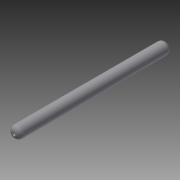
# Autodesk Inventor part: Pool Noodle Part2 (26x28 robot)
Saved by Autodesk Inventor 2014 SP1 (Build 180222100, 222)
## iProperties
Created: 2013-01-06
Part Number: Pool Noodle Part2 (26x28 robot)
Material: Generic
Document SubType Name: Modeling
Designer: Moses
Density: 0.0258246 g/cm^3
Mass: 45.1324 g
Surface Area: 1630.33 cm^2
Volume: 1747.66 cm^3
Appearance: Default
Author: Moses
Autodesk Inventor part; units mm, degrees
ref_plane "YZ Plane" through (0, 0, 0) normal (1, 0, 0) x (0, 1, 0)
ref_plane "XZ Plane" through (0, 0, 0) normal (0, 1, 0) x (-1, 0, 0)
ref_plane "XY Plane" through (0, 0, 0) normal (0, 0, 1) x (1, 0, 0)
sketch "Sketch1" plane through (0, 0, 0) normal (0, 0, 1) x (1, 0, 0)
  circle A0 centre (0, 0) radius 31.75
  circle A1 centre (0, 0) radius 9.525
  dimension "d0" = 63.5
  dimension "d1" = 19.05
  constraints: 2 centre point, 2 coincident
  measures "d0" diameter of A0
  measures "d1" diameter of A1
extrude "Extrusion1" add sketch "Sketch1" along normal blind 812.8
fillet "Fillet1" radius 25.4 2 edges at (-31.75, 0, 812.8) (-31.75, 0, 0)
body "Solid1"
